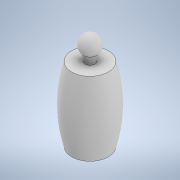
# Autodesk Inventor part: Tentalce Part
Saved by Autodesk Inventor 2021 (Build 250183000, 183)
## iProperties
Created: 2020-07-13
Part Number: Tentalce Part
Material: Generic
Document SubType Name: Modeling
Designer: saipr
Density: 1 g/cm^3
Appearance: Default
Author: saipr
Autodesk Inventor part; units mm, degrees
ref_plane "YZ Plane" through (0, 0, 0) normal (1, 0, 0) x (0, 1, 0)
ref_plane "XZ Plane" through (0, 0, 0) normal (0, 1, 0) x (-1, 0, 0)
ref_plane "XY Plane" through (0, 0, 0) normal (0, 0, 1) x (1, 0, 0)
sketch "Sketch1" plane through (0, 0, 0) normal (0, 0, 1) x (1, 0, 0)
  circle A0 centre (0, 0) radius 3.175
  line L0 (0, 0) -> (-2.2451, -2.2451)
  line L1 (0, 0) -> (2.2451, -2.2451)
  line L2 (0, 0) -> (3.175, 0)
  line L3 (0, 0) -> (0, -5.08)
  line L4 (0, -5.08) -> (1.651, -5.08)
  line L5 (1.651, -5.08) -> (-1.524, -5.08)
  arc A1 (-1.524, -5.08) -> (-2.2451, -2.2451) centre (-5.7114, -4.6359) ccw
  arc A2 (2.2451, -2.2451) -> (1.651, -5.08) centre (5.8874, -4.488) ccw
  line L6 (0, -5.08) -> (0, 3.175)
  line L7 (0, -5.08) -> (0, -30.48)
  line L8 (6.35, -30.48) -> (6.35, -5.08)
  line L9 (6.35, -5.08) -> (-6.35, -5.08)
  line L10 (-6.35, -5.08) -> (-6.35, -30.48)
  line L11 (-6.35, -30.48) -> (6.35, -5.08) construction
  line L12 (6.35, -30.48) -> (-6.35, -5.08) construction
  line L13 (0, -30.48) -> (0, -28.956)
  arc A3 (2.7853, -30.48) -> (-2.7853, -30.48) centre (0, -28.956) ccw
  line L14 (-6.35, -30.48) -> (-2.7853, -30.48)
  line L15 (2.7853, -30.48) -> (6.35, -30.48)
  arc A4 (6.35, -30.48) -> (6.35, -5.08) centre (-40.209, -17.78) ccw
  arc A5 (-6.35, -5.08) -> (-6.35, -30.48) centre (40.209, -17.78) ccw
  point P0 (0, -17.78)
  point P1 (0, -25.781)
  dimension "d0" = 6.35
  dimension "d1" = 90
  dimension "d2" = 45
  dimension "d3" = 5.08
  dimension "d6" = 25.4
  dimension "d7" = 12.7
  dimension "d8" = 1.524
  dimension "d9" = 6.35
  dimension "d11" = 48.26
  dimension "d12" = 48.26
  constraints: 32 end point, 14 point on circle, 6 centre point, 4 horizontal, 3 midpoint, 3 parallel, 3 vertical, 2 coincident, 2 perpendicular, 2 point on line
  measures "d0" diameter of A0
  measures "d1" angle of L0 L1
  measures "d2" angle of L2 L1
  measures "d3" distance of L0.start L3.end
  measures "d6" distance of L3.end L7.end
  measures "d7" distance of L9.end L8.end
  measures "d8" distance of L7.end L13.end
  measures "d9" diameter of A3
  measures "d11" radius of A4
  measures "d12" radius of A5
revolve "Revolution1" add sketch "Sketch1" angle 360 about axis through (0, -5.08, 0) along (0, -1, 0) contours L2 L6 A0 | A0 L1 L2 | A2 L4 L3 A0 | A0 L3 L1 | L9 L8 L15 A3 L7 L4 | A4 L8
sketch "Sketch2" plane through (0, -30.48, 0) normal (0, -1, 0) x (1, 0, 0)
  circle A0 centre (0, 0) radius 6.35
  dimension "d15" = 12.7
  constraints: 1 centre point, 1 coincident
  measures "d15" diameter of A0
body "Solid1"
